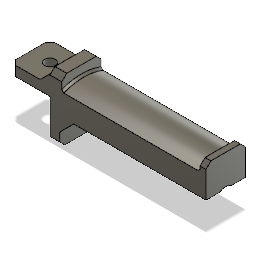
_simple_spool_mount.738eed80-4869-4e51-b167-2cb4ad1de5a5 (Autodesk Fusion 360 design; units mm, degrees)
Autodesk Fusion 360 part; units mm, degrees
note: some values were not read from the file. Set by a fixed rule: which sketch regions a step uses.
sketch "Sketch1" plane through (0, 0, 0) normal (0, 0, 1) x (1, 0, 0)
  line L0 (10, -10) -> (10, 10)
  line L1 (10, 10) -> (-10, 10)
  line L2 (-10, 10) -> (10, 10)
  line L3 (10, 15) -> (-10, 15)
  line L4 (-10, 15) -> (-10, 10)
  line L5 (10, 10) -> (10, -10)
  line L6 (10, -10) -> (15, -10)
  line L7 (15, -10) -> (15, 4)
  line L8 (13, 22) -> (10, 22)
  line L9 (10, 22) -> (10, 15)
  line L10 (13, 22) -> (16, 22)
  line L11 (16, 22) -> (16, 4)
  line L12 (16, 4) -> (15, 4)
  constraint vertical L0
  constraint horizontal L1
  constraint horizontal L2
  constraint horizontal L3
  constraint vertical L4
  constraint vertical L5
  constraint horizontal L6
  constraint vertical L7
  constraint horizontal L8
  constraint vertical L9
  constraint horizontal L10
  constraint vertical L11
  constraint horizontal L12
extrude "Extrude9" add sketch "Sketch1" along normal blind 20
sketch "Sketch10" plane through (0, 15, 0) normal (0, 1, 0) x (-1, 0, 0)
  line L0 (-10, 0) -> (10, 0)
  line L1 (10, 0) -> (10, 20)
  line L2 (10, 20) -> (-10, 20)
  line L3 (-10, 20) -> (-10, 0)
  circle A0 centre (0, 10) radius 2.75
  dimension "d34" = 5.5
  measures "d34" diameter of A0
extrude "Extrude10" cut sketch "Sketch10" against normal blind 5 contours A0
sketch "Sketch11" plane through (10, 0, 0) normal (-1, 0, 0) x (0, 0, 1)
  line L0 (0, 10) -> (0, -10)
  line L1 (0, -10) -> (20, -10)
  line L2 (20, -10) -> (20, 10)
  line L3 (20, 10) -> (0, 10)
  circle A0 centre (10, 0) radius 2.75
  dimension "d37" = 5.5
  measures "d37" diameter of A0
extrude "Extrude11" cut sketch "Sketch11" against normal blind 5 contours A0
sketch "Sketch12" plane through (16, 0, 0) normal (1, 0, 0) x (0, 0, -1)
  line L0 (0, 4) -> (0, 22)
  line L1 (0, 22) -> (-20, 22)
  line L2 (-20, 22) -> (-20, 4)
  line L3 (-20, 4) -> (0, 4)
  line L4 (0, -10) -> (-20, -10)
  arc A0 (0, 15.0799) -> (-20, 15.0799) centre (-10, -10) ccw
  constraint midpoint A0.centre L4
  constraint coincident L2 A0.end
  constraint coincident L0 A0.start
extrude "Extrude12" add sketch "Sketch12" along normal blind 70 contours L0 L2 L3 A0
sketch "Sketch13" plane through (86, 0, 0) normal (1, 0, 0) x (0, 0, -1)
  arc A0 (0, 15.0799) -> (-20, 15.0799) centre (-10, -10) ccw
  line L0 (-20, 15.0799) -> (-20, 4)
  line L1 (-20, 4) -> (0, 4)
  line L2 (0, 4) -> (0, 15.0799)
  line L3 (-20, 15.0799) -> (-20, 20.0799)
  line L4 (0, 15.0799) -> (0, 20.0799)
  line L5 (0, 20.0799) -> (-20, 20.0799)
  dimension "d42" = 5
  dimension "d43" = 5
  constraint coincident A0.end L0.start
  constraint parallel L0 L3
  constraint coincident A0.start L2.end
  constraint parallel L2 L4
  measures "d42" distance of A0.end L3.end
  measures "d43" distance of A0.start L4.end
extrude "Extrude13" add sketch "Sketch13" along normal blind 3
chamfer "Chamfer6" distance 1 angle 45 2 edges at (16, 17, 10) (86, 17, 10)
chamfer "Chamfer8" distance 2.5 angle 45 4 edges at (-10, 12.5, 20) (-10, 12.5, 0) (12.5, -10, 20) (12.5, -10, 0)
chamfer "Chamfer9" distance 2.5 angle 45 4 edges at (13, 22, 20) (87.5, 20.0799, 20) (13, 22, 0) (87.5, 20.0799, 0)
sketch "Sketch14" plane through (15, 0, 0) normal (1, 0, 0) x (0, 0, -1)
  line L0 (-2.5, -10) -> (0, -7.5)
  line L1 (0, -7.5) -> (0, 4)
  line L2 (-20, 4) -> (-20, -7.5)
  line L3 (-20, -7.5) -> (-17.5, -10)
  line L4 (-17.5, -10) -> (-2.5, -10)
  circle A0 centre (-10, 0) radius 5
  circle A1 centre (-10, 0) radius 2.75
  line L5 (0, 4) -> (-20, 4)
  dimension "d50" = 10
  measures "d50" diameter of A0
extrude "Extrude14" cut sketch "Sketch14" along normal blind 100 contours A0 L5 picked at (-10.7998, 4.1289)
chamfer "Chamfer10" distance 7 angle 45 2 edges at (15, 4, 3.5) (15, 4, 16.5)
chamfer "Chamfer11" distance 5 angle 45 1 edges at (10, 15, 10)
